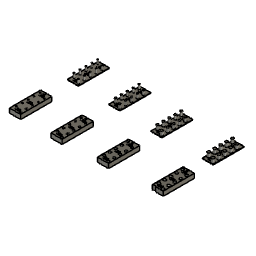
3DHoles And Pins Kit v6 (Autodesk Fusion 360 design; units mm, degrees)
Autodesk Fusion 360 part; units mm, degrees
sketch "Schizzo1" plane through (0, 0, 0) normal (0, 0, 1) x (1, 0, 0)
  line L0 (-82.079, 85.7376) -> (-57.079, 85.7376)
  line L1 (-57.079, 85.7376) -> (-57.079, 15.7376)
  line L2 (-57.079, 15.7376) -> (-82.079, 15.7376)
  line L3 (-82.079, 15.7376) -> (-82.079, 85.7376)
  line L4 (-77.579, 85.7376) -> (-77.579, 15.7376) construction
  line L5 (-69.579, 85.7376) -> (-69.579, 15.7376) construction
  line L6 (-61.579, 85.7376) -> (-61.579, 15.7376) construction
  line L7 (-82.079, 79.7376) -> (-57.079, 79.7376) construction
  line L8 (-82.079, 73.071) -> (-57.079, 73.071) construction
  line L9 (-82.079, 66.4043) -> (-57.079, 66.4043) construction
  line L10 (-82.079, 59.7376) -> (-57.079, 59.7376) construction
  line L11 (-82.079, 53.071) -> (-57.079, 53.071) construction
  line L12 (-82.079, 46.4043) -> (-57.079, 46.4043) construction
  line L13 (-82.079, 39.7376) -> (-57.079, 39.7376) construction
  line L14 (-82.079, 33.071) -> (-57.079, 33.071) construction
  line L15 (-82.079, 26.4043) -> (-57.079, 26.4043) construction
  line L16 (-82.079, 19.7376) -> (-57.079, 19.7376) construction
  circle A0 centre (-77.579, 79.7376) radius 2.5
  circle A1 centre (-77.579, 66.4043) radius 2.6
  circle A2 centre (-61.579, 73.071) radius 2.55
  circle A3 centre (-77.579, 53.071) radius 2.7
  circle A4 centre (-77.579, 39.7376) radius 2.8
  circle A5 centre (-77.579, 26.4043) radius 2.9
  circle A6 centre (-61.579, 59.7376) radius 2.65
  circle A7 centre (-61.579, 46.4043) radius 2.75
  circle A8 centre (-61.579, 33.071) radius 2.85
  circle A9 centre (-61.579, 19.7376) radius 2.95
  circle A10 centre (-61.579, -73.5957) radius 2.75
  line L17 (-82.079, -86.929) -> (-57.079, -86.929) construction
  line L18 (-57.079, -34.2624) -> (-57.079, -104.2624)
  line L19 (-57.079, -104.2624) -> (-82.079, -104.2624)
  line L20 (-61.579, -34.2624) -> (-61.579, -104.2624) construction
  line L21 (-82.079, -34.2624) -> (-57.079, -34.2624)
  circle A11 centre (-77.579, -40.2624) radius 2.5
  circle A12 centre (-61.579, -46.929) radius 2.55
  line L22 (-82.079, -80.2624) -> (-57.079, -80.2624) construction
  circle A13 centre (-61.579, -86.929) radius 2.85
  line L23 (-82.079, -104.2624) -> (-82.079, -34.2624)
  line L24 (-69.579, -34.2624) -> (-69.579, -104.2624) construction
  line L25 (-77.579, -34.2624) -> (-77.579, -104.2624) construction
  circle A14 centre (-77.579, -80.2624) radius 2.8
  circle A15 centre (-77.579, -66.929) radius 2.7
  line L26 (-82.079, -100.2624) -> (-57.079, -100.2624) construction
  line L27 (-82.079, -93.5957) -> (-57.079, -93.5957) construction
  line L28 (-82.079, -53.5957) -> (-57.079, -53.5957) construction
  line L29 (-82.079, -66.929) -> (-57.079, -66.929) construction
  circle A16 centre (-61.579, -60.2624) radius 2.65
  line L30 (-82.079, -46.929) -> (-57.079, -46.929) construction
  line L31 (-82.079, -40.2624) -> (-57.079, -40.2624) construction
  circle A17 centre (-77.579, -53.5957) radius 2.6
  line L32 (-82.079, -73.5957) -> (-57.079, -73.5957) construction
  circle A18 centre (-77.579, -93.5957) radius 2.9
  line L33 (-82.079, -60.2624) -> (-57.079, -60.2624) construction
  circle A19 centre (-61.579, -100.2624) radius 2.95
  line L34 (28.5016, 20.6114) -> (28.5016, 90.6114)
  circle A20 centre (33.0016, 84.6114) radius 3
  line L35 (28.5016, 24.6114) -> (53.5016, 24.6114) construction
  circle A21 centre (49.0016, 77.9447) radius 3.05
  line L36 (28.5016, 37.9447) -> (53.5016, 37.9447) construction
  line L37 (28.5016, 57.9447) -> (53.5016, 57.9447) construction
  line L38 (41.0016, 90.6114) -> (41.0016, 20.6114) construction
  line L39 (33.0016, 90.6114) -> (33.0016, 20.6114) construction
  line L40 (53.5016, 90.6114) -> (53.5016, 20.6114)
  circle A22 centre (49.0016, 51.2781) radius 3.25
  line L41 (28.5016, 51.2781) -> (53.5016, 51.2781) construction
  line L42 (28.5016, 71.2781) -> (53.5016, 71.2781) construction
  line L43 (28.5016, 84.6114) -> (53.5016, 84.6114) construction
  circle A23 centre (49.0016, 64.6114) radius 3.15
  circle A24 centre (49.0016, 24.6114) radius 3.45
  circle A25 centre (33.0016, 71.2781) radius 3.1
  line L44 (49.0016, 90.6114) -> (49.0016, 20.6114) construction
  line L45 (53.5016, 20.6114) -> (28.5016, 20.6114)
  line L46 (28.5016, 90.6114) -> (53.5016, 90.6114)
  circle A26 centre (33.0016, 57.9447) radius 3.2
  line L47 (28.5016, 44.6114) -> (53.5016, 44.6114) construction
  line L48 (28.5016, 77.9447) -> (53.5016, 77.9447) construction
  circle A27 centre (33.0016, 44.6114) radius 3.3
  circle A28 centre (49.0016, 37.9447) radius 3.35
  circle A29 centre (33.0016, 31.2781) radius 3.4
  line L49 (28.5016, 64.6114) -> (53.5016, 64.6114) construction
  line L50 (28.5016, 31.2781) -> (53.5016, 31.2781) construction
  line L51 (33.3177, -92.6248) -> (58.3177, -92.6248) construction
  line L52 (58.3177, -96.6248) -> (33.3177, -96.6248)
  line L53 (53.8177, -26.6248) -> (53.8177, -96.6248) construction
  line L54 (33.3177, -85.9581) -> (58.3177, -85.9581) construction
  line L55 (33.3177, -72.6248) -> (58.3177, -72.6248) construction
  circle A30 centre (37.8177, -85.9581) radius 3.4
  circle A31 centre (53.8177, -39.2914) radius 3.05
  circle A32 centre (37.8177, -45.9581) radius 3.1
  line L56 (33.3177, -45.9581) -> (58.3177, -45.9581) construction
  circle A33 centre (53.8177, -79.2914) radius 3.35
  circle A34 centre (37.8177, -32.6248) radius 3
  circle A35 centre (37.8177, -59.2914) radius 3.2
  line L57 (33.3177, -26.6248) -> (58.3177, -26.6248)
  line L58 (33.3177, -59.2914) -> (58.3177, -59.2914) construction
  circle A36 centre (53.8177, -52.6248) radius 3.15
  line L59 (33.3177, -79.2914) -> (58.3177, -79.2914) construction
  line L60 (33.3177, -52.6248) -> (58.3177, -52.6248) construction
  circle A37 centre (37.8177, -72.6248) radius 3.3
  circle A38 centre (53.8177, -92.6248) radius 3.45
  line L61 (33.3177, -65.9581) -> (58.3177, -65.9581) construction
  line L62 (33.3177, -32.6248) -> (58.3177, -32.6248) construction
  line L63 (33.3177, -39.2914) -> (58.3177, -39.2914) construction
  line L64 (37.8177, -26.6248) -> (37.8177, -96.6248) construction
  line L65 (33.3177, -96.6248) -> (33.3177, -26.6248)
  circle A39 centre (53.8177, -65.9581) radius 3.25
  line L66 (45.8177, -26.6248) -> (45.8177, -96.6248) construction
  line L67 (58.3177, -26.6248) -> (58.3177, -96.6248)
  line L68 (-181.4984, 44.6114) -> (-156.4984, 44.6114) construction
  circle A40 centre (-176.9984, 31.2781) radius 2.4
  line L69 (-156.4984, 20.6114) -> (-181.4984, 20.6114)
  circle A41 centre (-160.9984, 24.6114) radius 2.45
  line L70 (-181.4984, 51.2781) -> (-156.4984, 51.2781) construction
  circle A42 centre (-176.9984, 44.6114) radius 2.3
  line L71 (-181.4984, 37.9447) -> (-156.4984, 37.9447) construction
  line L72 (-181.4984, 31.2781) -> (-156.4984, 31.2781) construction
  line L73 (-160.9984, 90.6114) -> (-160.9984, 20.6114) construction
  circle A43 centre (-160.9984, 37.9447) radius 2.35
  line L74 (-181.4984, 90.6114) -> (-156.4984, 90.6114)
  circle A44 centre (-160.9984, 64.6114) radius 2.15
  line L75 (-181.4984, 57.9447) -> (-156.4984, 57.9447) construction
  line L76 (-181.4984, 71.2781) -> (-156.4984, 71.2781) construction
  line L77 (-181.4984, 84.6114) -> (-156.4984, 84.6114) construction
  line L78 (-168.9984, 90.6114) -> (-168.9984, 20.6114) construction
  line L79 (-156.4984, 90.6114) -> (-156.4984, 20.6114)
  line L80 (-176.9984, 90.6114) -> (-176.9984, 20.6114) construction
  line L81 (-181.4984, 20.6114) -> (-181.4984, 90.6114)
  circle A45 centre (-160.9984, 51.2781) radius 2.25
  circle A46 centre (-176.9984, 84.6114) radius 2
  line L82 (-181.4984, 77.9447) -> (-156.4984, 77.9447) construction
  line L83 (-181.4984, 24.6114) -> (-156.4984, 24.6114) construction
  circle A47 centre (-176.9984, 57.9447) radius 2.2
  circle A48 centre (-160.9984, 77.9447) radius 2.05
  line L84 (-181.4984, 64.6114) -> (-156.4984, 64.6114) construction
  circle A49 centre (-176.9984, 71.2781) radius 2.1
  line L85 (-181.4984, -78.7219) -> (-156.4984, -78.7219) construction
  line L86 (-181.4984, -45.3886) -> (-156.4984, -45.3886) construction
  line L87 (-181.4984, -92.0553) -> (-156.4984, -92.0553) construction
  circle A50 centre (-176.9984, -98.7219) radius 2.4
  circle A51 centre (-176.9984, -85.3886) radius 2.3
  circle A52 centre (-160.9984, -92.0553) radius 2.35
  line L88 (-156.4984, -109.3886) -> (-181.4984, -109.3886)
  line L89 (-176.9984, -39.3886) -> (-176.9984, -109.3886) construction
  line L90 (-181.4984, -52.0553) -> (-156.4984, -52.0553) construction
  line L91 (-181.4984, -105.3886) -> (-156.4984, -105.3886) construction
  line L92 (-181.4984, -109.3886) -> (-181.4984, -39.3886)
  line L93 (-156.4984, -39.3886) -> (-156.4984, -109.3886)
  circle A53 centre (-176.9984, -72.0553) radius 2.2
  line L94 (-160.9984, -39.3886) -> (-160.9984, -109.3886) construction
  line L95 (-168.9984, -39.3886) -> (-168.9984, -109.3886) construction
  circle A54 centre (-160.9984, -78.7219) radius 2.25
  circle A55 centre (-160.9984, -52.0553) radius 2.05
  circle A56 centre (-176.9984, -45.3886) radius 2
  line L96 (-181.4984, -39.3886) -> (-156.4984, -39.3886)
  line L97 (-181.4984, -58.7219) -> (-156.4984, -58.7219) construction
  line L98 (-181.4984, -65.3886) -> (-156.4984, -65.3886) construction
  circle A57 centre (-176.9984, -58.7219) radius 2.1
  line L99 (-181.4984, -72.0553) -> (-156.4984, -72.0553) construction
  circle A58 centre (-160.9984, -65.3886) radius 2.15
  circle A59 centre (-160.9984, -105.3886) radius 2.45
  line L100 (-181.4984, -98.7219) -> (-156.4984, -98.7219) construction
  line L101 (-181.4984, -85.3886) -> (-156.4984, -85.3886) construction
  circle A60 centre (-272.0657, 86.4576) radius 1.5
  circle A61 centre (-256.0657, 66.4576) radius 1.65
  line L102 (-276.5657, 92.4576) -> (-251.5657, 92.4576)
  line L103 (-276.5657, 59.7909) -> (-251.5657, 59.7909) construction
  circle A62 centre (-272.0657, 73.1243) radius 1.6
  line L104 (-276.5657, 33.1243) -> (-251.5657, 33.1243) construction
  line L105 (-276.5657, 79.7909) -> (-251.5657, 79.7909) construction
  line L106 (-251.5657, 22.4576) -> (-276.5657, 22.4576)
  line L107 (-276.5657, 26.4576) -> (-251.5657, 26.4576) construction
  circle A63 centre (-256.0657, 39.7909) radius 1.85
  circle A64 centre (-272.0657, 33.1243) radius 1.9
  line L108 (-276.5657, 53.1243) -> (-251.5657, 53.1243) construction
  line L109 (-276.5657, 46.4576) -> (-251.5657, 46.4576) construction
  line L110 (-276.5657, 39.7909) -> (-251.5657, 39.7909) construction
  circle A65 centre (-256.0657, 26.4576) radius 1.95
  circle A66 centre (-272.0657, 46.4576) radius 1.8
  line L111 (-251.5657, 92.4576) -> (-251.5657, 22.4576)
  line L112 (-276.5657, 66.4576) -> (-251.5657, 66.4576) construction
  circle A67 centre (-256.0657, 53.1243) radius 1.75
  line L113 (-256.0657, 92.4576) -> (-256.0657, 22.4576) construction
  line L114 (-276.5657, 73.1243) -> (-251.5657, 73.1243) construction
  circle A68 centre (-272.0657, 59.7909) radius 1.7
  circle A69 centre (-256.0657, 79.7909) radius 1.55
  line L115 (-272.0657, 92.4576) -> (-272.0657, 22.4576) construction
  line L116 (-276.5657, 86.4576) -> (-251.5657, 86.4576) construction
  line L117 (-276.5657, 22.4576) -> (-276.5657, 92.4576)
  line L118 (-264.0657, 92.4576) -> (-264.0657, 22.4576) construction
  line L119 (-276.5657, -43.5424) -> (-251.5657, -43.5424) construction
  line L120 (-256.0657, -37.5424) -> (-256.0657, -107.5424) construction
  line L121 (-276.5657, -103.5424) -> (-251.5657, -103.5424) construction
  circle A70 centre (-256.0657, -103.5424) radius 1.95
  line L122 (-276.5657, -50.2091) -> (-251.5657, -50.2091) construction
  line L123 (-276.5657, -76.8757) -> (-251.5657, -76.8757) construction
  circle A71 centre (-272.0657, -56.8757) radius 1.6
  line L124 (-276.5657, -37.5424) -> (-251.5657, -37.5424)
  circle A72 centre (-256.0657, -76.8757) radius 1.75
  line L125 (-276.5657, -56.8757) -> (-251.5657, -56.8757) construction
  circle A73 centre (-256.0657, -63.5424) radius 1.65
  circle A74 centre (-256.0657, -50.2091) radius 1.55
  circle A75 centre (-272.0657, -70.2091) radius 1.7
  circle A76 centre (-272.0657, -43.5424) radius 1.5
  line L126 (-276.5657, -70.2091) -> (-251.5657, -70.2091) construction
  line L127 (-276.5657, -63.5424) -> (-251.5657, -63.5424) construction
  circle A77 centre (-272.0657, -83.5424) radius 1.8
  line L128 (-251.5657, -37.5424) -> (-251.5657, -107.5424)
  circle A78 centre (-272.0657, -96.8757) radius 1.9
  line L129 (-264.0657, -37.5424) -> (-264.0657, -107.5424) construction
  line L130 (-272.0657, -37.5424) -> (-272.0657, -107.5424) construction
  line L131 (-251.5657, -107.5424) -> (-276.5657, -107.5424)
  line L132 (-276.5657, -96.8757) -> (-251.5657, -96.8757) construction
  line L133 (-276.5657, -107.5424) -> (-276.5657, -37.5424)
  line L134 (-276.5657, -83.5424) -> (-251.5657, -83.5424) construction
  line L135 (-276.5657, -90.2091) -> (-251.5657, -90.2091) construction
  circle A79 centre (-256.0657, -90.2091) radius 1.85
  line L136 (33.3177, -98.6248) -> (58.3177, -98.6248) construction
  circle A80 centre (37.8177, -98.6248) radius 4
  dimension "d1" = 25
  dimension "d2" = 70
  dimension "d5" = 8
  dimension "d18" = 60
  dimension "d19" = 0
  dimension "d20" = 6
  dimension "d21" = 5
  dimension "d23" = 5
  dimension "d24" = 5.2
  dimension "d25" = 5.1
  dimension "d26" = 5.4
  dimension "d27" = 5.6
  dimension "d28" = 5.8
  dimension "d29" = 5
  dimension "d30" = 5.3
  dimension "d31" = 5.5
  dimension "d32" = 5
  dimension "d33" = 5.7
  dimension "d34" = 5.9
  dimension "d35" = 5
  dimension "d36" = 5
  dimension "d37" = 5
  dimension "d40" = 60
  dimension "d41" = 0
  dimension "d42" = 25
  dimension "d43" = 70
  dimension "d44" = 8
  dimension "d45" = 6
  dimension "d46" = 5
  dimension "d47" = 5.2
  dimension "d48" = 5.1
  dimension "d49" = 5.4
  dimension "d50" = 5.6
  dimension "d51" = 5.8
  dimension "d52" = 5.3
  dimension "d53" = 5.5
  dimension "d54" = 5.7
  dimension "d55" = 5.9
  dimension "d62" = 5
  dimension "d65" = 5
  dimension "d69" = 5
  dimension "d70" = 5
  dimension "d71" = 5
  dimension "d72" = 5
  dimension "d75" = 60
  dimension "d76" = 0
  dimension "d77" = 25
  dimension "d78" = 70
  dimension "d79" = 8
  dimension "d80" = 6
  dimension "d81" = 6
  dimension "d82" = 6.2
  dimension "d83" = 6.1
  dimension "d84" = 6.4
  dimension "d85" = 6.6
  dimension "d86" = 6.8
  dimension "d87" = 6.3
  dimension "d88" = 6.5
  dimension "d89" = 6.7
  dimension "d90" = 6.9
  dimension "d91" = 5
  dimension "d92" = 5
  dimension "d93" = 5
  dimension "d94" = 5
  dimension "d97" = 60
  dimension "d98" = 0
  dimension "d99" = 25
  dimension "d100" = 70
  dimension "d101" = 8
  dimension "d102" = 6
  dimension "d103" = 6
  dimension "d104" = 6.2
  dimension "d105" = 6.1
  dimension "d106" = 6.4
  dimension "d107" = 6.6
  dimension "d108" = 6.8
  dimension "d109" = 6.3
  dimension "d110" = 6.5
  dimension "d111" = 6.7
  dimension "d112" = 6.9
  dimension "d128" = 5
  dimension "d129" = 5
  dimension "d130" = 5
  dimension "d131" = 5
  dimension "d134" = 60
  dimension "d135" = 0
  dimension "d136" = 25
  dimension "d137" = 70
  dimension "d138" = 8
  dimension "d139" = 6
  dimension "d140" = 4
  dimension "d141" = 4.2
  dimension "d142" = 4.1
  dimension "d143" = 4.4
  dimension "d144" = 4.6
  dimension "d145" = 4.8
  dimension "d146" = 4.3
  dimension "d147" = 4.5
  dimension "d148" = 4.7
  dimension "d149" = 4.9
  dimension "d150" = 5
  dimension "d151" = 5
  dimension "d152" = 5
  dimension "d153" = 5
  dimension "d156" = 60
  dimension "d157" = 0
  dimension "d158" = 25
  dimension "d159" = 70
  dimension "d160" = 8
  dimension "d161" = 6
  dimension "d162" = 4
  dimension "d163" = 4.2
  dimension "d164" = 4.1
  dimension "d165" = 4.4
  dimension "d166" = 4.6
  dimension "d167" = 4.8
  dimension "d168" = 4.3
  dimension "d169" = 4.5
  dimension "d170" = 4.7
  dimension "d171" = 4.9
  dimension "d172" = 5
  dimension "d173" = 5
  dimension "d174" = 5
  dimension "d175" = 5
  dimension "d178" = 60
  dimension "d179" = 0
  dimension "d180" = 25
  dimension "d181" = 70
  dimension "d182" = 8
  dimension "d183" = 6
  dimension "d184" = 3
  dimension "d185" = 3.2
  dimension "d186" = 3.1
  dimension "d187" = 3.4
  dimension "d188" = 3.6
  dimension "d189" = 3.8
  dimension "d190" = 3.3
  dimension "d191" = 3.5
  dimension "d192" = 3.7
  dimension "d193" = 3.9
  dimension "d194" = 5
  dimension "d195" = 5
  dimension "d196" = 5
  dimension "d197" = 5
  dimension "d200" = 60
  dimension "d201" = 0
  dimension "d202" = 25
  dimension "d203" = 70
  dimension "d204" = 8
  dimension "d205" = 6
  dimension "d206" = 3
  dimension "d207" = 3.2
  dimension "d208" = 3.1
  dimension "d209" = 3.4
  dimension "d210" = 3.6
  dimension "d211" = 3.8
  dimension "d212" = 3.3
  dimension "d213" = 3.5
  dimension "d214" = 3.7
  dimension "d215" = 3.9
  dimension "d240" = 8
  dimension "d241" = 2
  text T0 "5" font "Arial" height 5 align centre spacing 1 along the path L7 letters at x, y, angle (-71.5214, 86.061, 0)
  text T1 ".10" font "Arial" height 5 align centre spacing 1 along the path L8 letters at x, y, angle (-74.4341, 79.3943, 0) (-72.4934, 79.3943, 0) (-68.6087, 79.3943, 0)
  text T2 ".50" font "Arial" height 5 align centre spacing 1 along the path L12 letters at x, y, angle (-74.4341, 52.7276, 0) (-72.4934, 52.7276, 0) (-68.6087, 52.7276, 0)
  text T3 ".10" font "Arial" height 5 align centre spacing 1 along the path L30 letters at x, y, angle (-74.4341, -40.6057, 0) (-72.4934, -40.6057, 0) (-68.6087, -40.6057, 0)
  text T4 "5" font "Arial" height 5 align centre spacing 1 along the path L31 letters at x, y, angle (-71.5214, -33.939, 0)
  text T5 ".50" font "Arial" height 5 align centre spacing 1 along the path L32 letters at x, y, angle (-74.4341, -67.2724, 0) (-72.4934, -67.2724, 0) (-68.6087, -67.2724, 0)
  text T6 ".90" font "Arial" height 5 align centre spacing 1 along the path L16 letters at x, y, angle (-74.4341, 26.061, 0) (-72.4934, 26.061, 0) (-68.6087, 26.061, 0)
  text T7 ".90" font "Arial" height 5 align centre spacing 1 along the path L26 letters at x, y, angle (-74.4341, -93.939, 0) (-72.4934, -93.939, 0) (-68.6087, -93.939, 0)
  text T8 ".90" font "Arial" height 5 align centre spacing 1 along the path L35 letters at x, y, angle (36.1465, 30.9347, 0) (38.0872, 30.9347, 0) (41.9719, 30.9347, 0)
  text T9 ".50" font "Arial" height 5 align centre spacing 1 along the path L41 letters at x, y, angle (36.1465, 57.6014, 0) (38.0872, 57.6014, 0) (41.9719, 57.6014, 0)
  text T10 "6" font "Arial" height 5 align centre spacing 1 along the path L43 letters at x, y, angle (39.0592, 90.9347, 0)
  text T11 ".10" font "Arial" height 5 align centre spacing 1 along the path L48 letters at x, y, angle (36.1465, 84.2681, 0) (38.0872, 84.2681, 0) (41.9719, 84.2681, 0)
  text T12 ".90" font "Arial" height 5 align centre spacing 1 along the path L51 letters at x, y, angle (40.9627, -86.3014, 0) (42.9033, -86.3014, 0) (46.788, -86.3014, 0)
  text T13 ".50" font "Arial" height 5 align centre spacing 1 along the path L61 letters at x, y, angle (40.9627, -59.6348, 0) (42.9033, -59.6348, 0) (46.788, -59.6348, 0)
  text T14 "6" font "Arial" height 5 align centre spacing 1 along the path L62 letters at x, y, angle (43.8754, -26.3014, 0)
  text T15 ".10" font "Arial" height 5 align centre spacing 1 along the path L63 letters at x, y, angle (40.9627, -32.9681, 0) (42.9033, -32.9681, 0) (46.788, -32.9681, 0)
  text T16 ".50" font "Arial" height 5 align centre spacing 1 along the path L70 letters at x, y, angle (-173.8535, 57.6014, 0) (-171.9128, 57.6014, 0) (-168.0281, 57.6014, 0)
  text T17 "4" font "Arial" height 5 align centre spacing 1 along the path L77 letters at x, y, angle (-170.9408, 90.9347, 0)
  text T18 ".10" font "Arial" height 5 align centre spacing 1 along the path L82 letters at x, y, angle (-173.8535, 84.2681, 0) (-171.9128, 84.2681, 0) (-168.0281, 84.2681, 0)
  text T19 ".90" font "Arial" height 5 align centre spacing 1 along the path L83 letters at x, y, angle (-173.8535, 30.9347, 0) (-171.9128, 30.9347, 0) (-168.0281, 30.9347, 0)
  text T20 ".50" font "Arial" height 5 align centre spacing 1 along the path L85 letters at x, y, angle (-173.8535, -72.3986, 0) (-171.9128, -72.3986, 0) (-168.0281, -72.3986, 0)
  text T21 "4" font "Arial" height 5 align centre spacing 1 along the path L86 letters at x, y, angle (-170.9408, -39.0653, 0)
  text T22 ".10" font "Arial" height 5 align centre spacing 1 along the path L90 letters at x, y, angle (-173.8535, -45.7319, 0) (-171.9128, -45.7319, 0) (-168.0281, -45.7319, 0)
  text T23 ".90" font "Arial" height 5 align centre spacing 1 along the path L91 letters at x, y, angle (-173.8535, -99.0653, 0) (-171.9128, -99.0653, 0) (-168.0281, -99.0653, 0)
  text T24 ".10" font "Arial" height 5 align centre spacing 1 along the path L105 letters at x, y, angle (-268.9207, 86.1143, 0) (-266.98, 86.1143, 0) (-263.0953, 86.1143, 0)
  text T25 ".90" font "Arial" height 5 align centre spacing 1 along the path L107 letters at x, y, angle (-268.9207, 32.7809, 0) (-266.98, 32.7809, 0) (-263.0953, 32.7809, 0)
  text T26 ".50" font "Arial" height 5 align centre spacing 1 along the path L108 letters at x, y, angle (-268.9207, 59.4476, 0) (-266.98, 59.4476, 0) (-263.0953, 59.4476, 0)
  text T27 "3" font "Arial" height 5 align centre spacing 1 along the path L116 letters at x, y, angle (-266.008, 92.7809, 0)
  text T28 "3" font "Arial" height 5 align centre spacing 1 along the path L119 letters at x, y, angle (-266.008, -37.2191, 0)
  text T29 ".90" font "Arial" height 5 align centre spacing 1 along the path L121 letters at x, y, angle (-268.9207, -97.2191, 0) (-266.98, -97.2191, 0) (-263.0953, -97.2191, 0)
  text T30 ".10" font "Arial" height 5 align centre spacing 1 along the path L122 letters at x, y, angle (-268.9207, -43.8857, 0) (-266.98, -43.8857, 0) (-263.0953, -43.8857, 0)
  text T31 ".50" font "Arial" height 5 align centre spacing 1 along the path L123 letters at x, y, angle (-268.9207, -70.5524, 0) (-266.98, -70.5524, 0) (-263.0953, -70.5524, 0)
  constraint horizontal L0
  constraint vertical L1
  constraint horizontal L2
  constraint vertical L3
  constraint coincident L0 L4.start
  constraint coincident L2 L4.end
  constraint perpendicular L2 L4
  constraint midpoint L0 L5.start
  constraint perpendicular L0 L5
  constraint symmetric L4.start L5 L6.start
  constraint symmetric L4.end L5 L6.end
  constraint midpoint L2 L5.end
  constraint coincident L3 L7.start
  constraint coincident L1 L7.end
  constraint perpendicular L1 L7
  constraint coincident L4 A0.centre
  constraint coincident L7 A0.centre
  constraint coincident L9 A1.centre
  constraint coincident L4 A1.centre
  constraint coincident L8 A2.centre
  constraint coincident L6 A2.centre
  constraint coincident L4 A3.centre
  constraint coincident L11 A3.centre
  constraint coincident L4 A4.centre
  constraint coincident L13 A4.centre
  constraint coincident L15 A5.centre
  constraint coincident L4 A5.centre
  constraint coincident L10 A6.centre
  constraint coincident L6 A6.centre
  constraint coincident L6 A7.centre
  constraint coincident L12 A7.centre
  constraint coincident L14 A8.centre
  constraint coincident L6 A8.centre
  constraint coincident L16 A9.centre
  constraint coincident L6 A9.centre
  constraint horizontal L21
  constraint vertical L18
  constraint horizontal L19
  constraint vertical L23
  constraint coincident L25.start L21
  constraint coincident L25.end L19
  constraint perpendicular L19 L25
  constraint midpoint L24.start L21
  constraint perpendicular L21 L24
  constraint symmetric L25.start L20.start L24
  constraint symmetric L25.end L20.end L24
  constraint midpoint L24.end L19
  constraint coincident L31.start L23
  constraint coincident L31.end L18
  constraint perpendicular L18 L31
  constraint coincident A11.centre L25
  constraint coincident A11.centre L31
  constraint coincident A17.centre L28
  constraint coincident A17.centre L25
  constraint coincident A12.centre L30
  constraint coincident A12.centre L20
  constraint coincident A15.centre L25
  constraint coincident A15.centre L29
  constraint coincident A14.centre L25
  constraint coincident A14.centre L22
  constraint coincident A18.centre L27
  constraint coincident A18.centre L25
  constraint coincident A16.centre L33
  constraint coincident A16.centre L20
  constraint coincident A10.centre L20
  constraint coincident A10.centre L32
  constraint coincident A13.centre L17
  constraint coincident A13.centre L20
  constraint coincident A19.centre L26
  constraint coincident A19.centre L20
  constraint horizontal L46
  constraint vertical L40
  constraint horizontal L45
  constraint vertical L34
  constraint coincident L39.start L46
  constraint coincident L39.end L45
  constraint perpendicular L39 L45
  constraint midpoint L38.start L46
  constraint perpendicular L38 L46
  constraint symmetric L44.start L39.start L38
  constraint symmetric L44.end L39.end L38
  constraint midpoint L38.end L45
  constraint coincident L43.start L34
  constraint coincident L43.end L40
  constraint perpendicular L40 L43
  constraint coincident A20.centre L39
  constraint coincident A20.centre L43
  constraint coincident A25.centre L42
  constraint coincident A25.centre L39
  constraint coincident A21.centre L48
  constraint coincident A21.centre L44
  constraint coincident A26.centre L39
  constraint coincident A26.centre L37
  constraint coincident A27.centre L39
  constraint coincident A27.centre L47
  constraint coincident A29.centre L50
  constraint coincident A29.centre L39
  constraint coincident A23.centre L49
  constraint coincident A23.centre L44
  constraint coincident A22.centre L44
  constraint coincident A22.centre L41
  constraint coincident A28.centre L36
  constraint coincident A28.centre L44
  constraint coincident A24.centre L35
  constraint coincident A24.centre L44
  constraint horizontal L57
  constraint vertical L67
  constraint horizontal L52
  constraint vertical L65
  constraint coincident L64.start L57
  constraint coincident L64.end L52
  constraint perpendicular L52 L64
  constraint midpoint L66.start L57
  constraint perpendicular L57 L66
  constraint symmetric L64.start L53.start L66
  constraint symmetric L64.end L53.end L66
  constraint midpoint L66.end L52
  constraint coincident L62.start L65
  constraint coincident L62.end L67
  constraint perpendicular L62 L67
  constraint coincident A34.centre L64
  constraint coincident A34.centre L62
  constraint coincident A32.centre L56
  constraint coincident A32.centre L64
  constraint coincident A31.centre L63
  constraint coincident A31.centre L53
  constraint coincident A35.centre L64
  constraint coincident A35.centre L58
  constraint coincident A37.centre L64
  constraint coincident A37.centre L55
  constraint coincident A30.centre L54
  constraint coincident A30.centre L64
  constraint coincident A36.centre L60
  constraint coincident A36.centre L53
  constraint coincident A39.centre L53
  constraint coincident A39.centre L61
  constraint coincident A33.centre L59
  constraint coincident A33.centre L53
  constraint coincident A38.centre L51
  constraint coincident A38.centre L53
  constraint horizontal L74
  constraint vertical L79
  constraint horizontal L69
  constraint vertical L81
  constraint coincident L80.start L74
  constraint coincident L80.end L69
  constraint perpendicular L69 L80
  constraint midpoint L78.start L74
  constraint perpendicular L74 L78
  constraint symmetric L80.start L73.start L78
  constraint symmetric L80.end L73.end L78
  constraint midpoint L78.end L69
  constraint coincident L77.start L81
  constraint coincident L77.end L79
  constraint perpendicular L77 L79
  constraint coincident A46.centre L80
  constraint coincident A46.centre L77
  constraint coincident A49.centre L76
  constraint coincident A49.centre L80
  constraint coincident A48.centre L82
  constraint coincident A48.centre L73
  constraint coincident A47.centre L80
  constraint coincident A47.centre L75
  constraint coincident A42.centre L80
  constraint coincident A42.centre L68
  constraint coincident A40.centre L72
  constraint coincident A40.centre L80
  constraint coincident A44.centre L84
  constraint coincident A44.centre L73
  constraint coincident A45.centre L73
  constraint coincident A45.centre L70
  constraint coincident A43.centre L71
  constraint coincident A43.centre L73
  constraint coincident A41.centre L83
  constraint coincident A41.centre L73
  constraint horizontal L96
  constraint vertical L93
  constraint horizontal L88
  constraint vertical L92
  constraint coincident L89.start L96
  constraint coincident L89.end L88
  constraint perpendicular L88 L89
  constraint midpoint L95.start L96
  constraint perpendicular L95 L96
  constraint symmetric L89.start L94.start L95
  constraint symmetric L94.end L89.end L95
  constraint midpoint L95.end L88
  constraint coincident L86.start L92
  constraint coincident L86.end L93
  constraint perpendicular L86 L93
  constraint coincident A56.centre L89
  constraint coincident A56.centre L86
  constraint coincident A57.centre L97
  constraint coincident A57.centre L89
  constraint coincident A55.centre L90
  constraint coincident A55.centre L94
  constraint coincident A53.centre L89
  constraint coincident A53.centre L99
  constraint coincident A51.centre L89
  constraint coincident A51.centre L101
  constraint coincident A50.centre L100
  constraint coincident A50.centre L89
  constraint coincident A58.centre L98
  constraint coincident A58.centre L94
  constraint coincident A54.centre L94
  constraint coincident A54.centre L85
  constraint coincident A52.centre L87
  constraint coincident A52.centre L94
  constraint coincident A59.centre L91
  constraint coincident A59.centre L94
  constraint horizontal L102
  constraint vertical L111
  constraint horizontal L106
  constraint vertical L117
  constraint coincident L115.start L102
  constraint coincident L115.end L106
  constraint perpendicular L106 L115
  constraint midpoint L118.start L102
  constraint perpendicular L102 L118
  constraint symmetric L115.start L113.start L118
  constraint symmetric L113.end L115.end L118
  constraint midpoint L118.end L106
  constraint coincident L116.start L117
  constraint coincident L116.end L111
  constraint perpendicular L111 L116
  constraint coincident A60.centre L115
  constraint coincident A60.centre L116
  constraint coincident A62.centre L114
  constraint coincident A62.centre L115
  constraint coincident A69.centre L105
  constraint coincident A69.centre L113
  constraint coincident A68.centre L115
  constraint coincident A68.centre L103
  constraint coincident A66.centre L115
  constraint coincident A66.centre L109
  constraint coincident A64.centre L104
  constraint coincident A64.centre L115
  constraint coincident A61.centre L112
  constraint coincident A61.centre L113
  constraint coincident A67.centre L113
  constraint coincident A67.centre L108
  constraint coincident A63.centre L110
  constraint coincident A63.centre L113
  constraint coincident A65.centre L107
  constraint coincident A65.centre L113
  constraint horizontal L124
  constraint vertical L128
  constraint horizontal L131
  constraint vertical L133
  constraint coincident L130.start L124
  constraint coincident L130.end L131
  constraint perpendicular L130 L131
  constraint midpoint L129.start L124
  constraint perpendicular L124 L129
  constraint symmetric L130.start L120.start L129
  constraint symmetric L120.end L130.end L129
  constraint midpoint L129.end L131
  constraint coincident L119.start L133
  constraint coincident L119.end L128
  constraint perpendicular L119 L128
  constraint coincident A76.centre L130
  constraint coincident A76.centre L119
  constraint coincident A71.centre L125
  constraint coincident A71.centre L130
  constraint coincident A74.centre L122
  constraint coincident A74.centre L120
  constraint coincident A75.centre L130
  constraint coincident A75.centre L126
  constraint coincident A77.centre L130
  constraint coincident A77.centre L134
  constraint coincident A78.centre L132
  constraint coincident A78.centre L130
  constraint coincident A73.centre L127
  constraint coincident A73.centre L120
  constraint coincident A72.centre L120
  constraint coincident A72.centre L123
  constraint coincident A79.centre L135
  constraint coincident A79.centre L120
  constraint coincident A70.centre L121
  constraint coincident A70.centre L120
  constraint perpendicular L67 L136
  constraint coincident L136 A80.centre
  constraint coincident L64 A80.centre
  measures "d1" distance of L0.start L0.end
  measures "d2" distance of L0.start L2.end
  measures "d5" distance of L4 L5
  measures "d20" distance of L0 L7
  measures "d23" diameter of A0
  measures "d24" diameter of A1
  measures "d25" diameter of A2
  measures "d26" diameter of A3
  measures "d27" diameter of A4
  measures "d28" diameter of A5
  measures "d30" diameter of A6
  measures "d31" diameter of A7
  measures "d33" diameter of A8
  measures "d34" diameter of A9
  measures "d42" distance of L18.start L21.start
  measures "d43" distance of L19.end L21.start
  measures "d44" distance of L24 L25
  measures "d45" distance of L21 L31
  measures "d46" diameter of A11
  measures "d47" diameter of A17
  measures "d48" diameter of A12
  measures "d49" diameter of A15
  measures "d50" diameter of A14
  measures "d51" diameter of A18
  measures "d52" diameter of A16
  measures "d53" diameter of A10
  measures "d54" diameter of A13
  measures "d55" diameter of A19
  measures "d77" distance of L40.start L34.end
  measures "d78" distance of L34.end L34.start
  measures "d79" distance of L38 L39
  measures "d80" distance of L43 L46
  measures "d81" diameter of A20
  measures "d82" diameter of A25
  measures "d83" diameter of A21
  measures "d84" diameter of A26
  measures "d85" diameter of A27
  measures "d86" diameter of A29
  measures "d87" diameter of A23
  measures "d88" diameter of A22
  measures "d89" diameter of A28
  measures "d90" diameter of A24
  measures "d99" distance of L57.end L57.start
  measures "d100" distance of L52.end L57.start
  measures "d101" distance of L64 L66
  measures "d102" distance of L57 L62
  measures "d103" diameter of A34
  measures "d104" diameter of A32
  measures "d105" diameter of A31
  measures "d106" diameter of A35
  measures "d107" diameter of A37
  measures "d108" diameter of A30
  measures "d109" diameter of A36
  measures "d110" diameter of A39
  measures "d111" diameter of A33
  measures "d112" diameter of A38
  measures "d136" distance of L74.end L74.start
  measures "d137" distance of L69.end L74.start
  measures "d138" distance of L78 L80
  measures "d139" distance of L74 L77
  measures "d140" diameter of A46
  measures "d141" diameter of A49
  measures "d142" diameter of A48
  measures "d143" diameter of A47
  measures "d144" diameter of A42
  measures "d145" diameter of A40
  measures "d146" diameter of A44
  measures "d147" diameter of A45
  measures "d148" diameter of A43
  measures "d149" diameter of A41
  measures "d158" distance of L92.end L93.start
  measures "d159" distance of L88.end L92.end
  measures "d160" distance of L89 L95
  measures "d161" distance of L86 L96
  measures "d162" diameter of A56
  measures "d163" diameter of A57
  measures "d164" diameter of A55
  measures "d165" diameter of A53
  measures "d166" diameter of A51
  measures "d167" diameter of A50
  measures "d168" diameter of A58
  measures "d169" diameter of A54
  measures "d170" diameter of A52
  measures "d171" diameter of A59
  measures "d180" distance of L102.start L102.end
  measures "d181" distance of L106.end L102.start
  measures "d182" distance of L115 L118
  measures "d183" distance of L102 L116
  measures "d184" diameter of A60
  measures "d185" diameter of A62
  measures "d186" diameter of A69
  measures "d187" diameter of A68
  measures "d188" diameter of A66
  measures "d189" diameter of A64
  measures "d190" diameter of A61
  measures "d191" diameter of A67
  measures "d192" diameter of A63
  measures "d193" diameter of A65
  measures "d202" distance of L124.start L124.end
  measures "d203" distance of L131.end L124.start
  measures "d204" distance of L129 L130
  measures "d205" distance of L119 L124
  measures "d206" diameter of A76
  measures "d207" diameter of A71
  measures "d208" diameter of A74
  measures "d209" diameter of A75
  measures "d210" diameter of A77
  measures "d211" diameter of A78
  measures "d212" diameter of A73
  measures "d213" diameter of A72
  measures "d214" diameter of A79
  measures "d215" diameter of A70
  measures "d240" diameter of A80
  measures "d241" distance of L52 L136
extrude "Estrusione1" add sketch "Schizzo1" along normal blind 0.8 contours L0 L1 L2 L3 makes body 1
extrude "Estrusione2" add sketch "Schizzo1" along normal blind 10 contours A0 | A1 | A2 | A3 | A4 | A5 | A6 | A7 | A8 | A9 bodies 1
extrude "Estrusione3" add sketch "Schizzo1" along normal blind 1.2 text T0 T1 T2 T6 bodies 1
extrude "Estrusione8" add sketch "Schizzo1" along normal blind 0.8 separate body contours L34 L40 L45 L46 makes body 2
extrude "Estrusione9" add sketch "Schizzo1" along normal blind 10 contours A20 | A21 | A22 | A23 | A24 | A25 | A26 | A27 | A28 | A29 bodies 2
extrude "Estrusione11" add sketch "Schizzo1" along normal blind 0.4 from surface at 0.8 text T8 T9 T11 T10 bodies 2
extrude "Estrusione4" add sketch "Schizzo1" along normal blind 10 separate body contours L18 L19 L21 L23 makes body 3
extrude "Estrusione5" add sketch "Schizzo1" along normal blind 0.4 from surface at 10 text T7 T5 T3 T4 bodies 3
extrude "Estrusione6" add sketch "Schizzo1" along normal blind 10 separate body contours L52 L57 L65 L67 A80 makes body 4
extrude "Estrusione7" add sketch "Schizzo1" along normal blind 0.5 from surface at 10 text T12 T13 T15 T14 bodies 4
extrude "Estrusione12" add sketch "Schizzo1" along normal blind 0.8 separate body contours L102 L106 L111 L117 makes body 5
extrude "Estrusione13" add sketch "Schizzo1" along normal blind 10 contours A60 | A61 | A62 | A63 | A64 | A65 | A66 | A67 | A68 | A69 bodies 5
extrude "Estrusione14" add sketch "Schizzo1" along normal blind 0.4 from surface at 0.8 text T27 T24 T26 T25 bodies 5
extrude "Estrusione15" add sketch "Schizzo1" along normal blind 10 separate body contours L124 L128 L131 L133 makes body 6
extrude "Estrusione16" add sketch "Schizzo1" along normal blind 0.4 from surface at 10 text T29 T31 T30 T28 bodies 6
extrude "Estrusione17" add sketch "Schizzo1" along normal blind 0.8 separate body contours L69 L74 L79 L81 makes body 7
extrude "Estrusione18" add sketch "Schizzo1" along normal blind 10 contours A40 | A41 | A42 | A43 | A44 | A45 | A46 | A47 | A48 | A49 bodies 7
extrude "Estrusione19" add sketch "Schizzo1" along normal blind 0.4 from surface at 0.8 text T17 T18 T16 T19 bodies 7
extrude "Estrusione20" add sketch "Schizzo1" along normal blind 10 separate body contours L88 L92 L93 L96 makes body 8
extrude "Estrusione21" add sketch "Schizzo1" along normal blind 0.4 from surface at 10 text T21 T22 T20 T23 bodies 8
equation "d82 = d81 + 0.2 mm"
equation "d83 = d81 + 0.1 mm"
equation "d84 = d81 + 0.4 mm"
equation "d85 = d81 + 0.6 mm"
equation "d86 = d81 + 0.8 mm"
equation "d87 = d81 + 0.3 mm"
equation "d88 = d81 + 0.5 mm"
equation "d89 = d81 + 0.7 mm"
equation "d90 = d81 + 0.9 mm"
equation "d104 = d81 + 0.2 mm"
equation "d105 = d81 + 0.1 mm"
equation "d106 = d81 + 0.4 mm"
equation "d107 = d81 + 0.6 mm"
equation "d108 = d81 + 0.8 mm"
equation "d109 = d81 + 0.3 mm"
equation "d110 = d81 + 0.5 mm"
equation "d111 = d81 + 0.7 mm"
equation "d112 = d81 + 0.9 mm"
named bodies: "5 mm stud", "5 mm hole", "6 mm hole", "6 mm stud", "3 mm stud", "3 mm hole", "4 mm stud", "4 mm hole"
